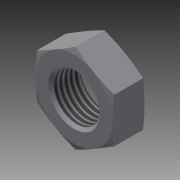
# Autodesk Inventor part: D-98
Saved by Autodesk Inventor 2014 SP2 (Build 180246200, 246)
## iProperties
Created: 2019-01-30
Part Number: D-98
Material: Generic
Catalog Web Link: www.cadenas.de
Description: Mounting Nut for Original Line Cylinders-
Vendor: BIMBA
Document SubType Name: Modeling
Designer: psadmin
Manufacturer: BIMBA
Mass: 1.65694 g
Surface Area: 11.8363 cm^2
Volume: 1.65694 cm^3
Density: 1 g/cm^3
Appearance: PSOLRGB-191-191-191
Category: PARTsolutions
Company: BIMBA
Title: D-98
Author: Cadenas PARTsolutions
PSOL_IDENT_0: {$CADENAS_DATA\23d-libs\bimba\bimba\bimba_imperial\bimba_full_line\original_line_cylinders\accessori
PSOL_IDENT_1: es\mounting_nut.prj},185 {VTYP=3D},{NB=D-98},{LINA=D-98},{NN=Mounting Nut for Original Line Cylinder
PSOL_IDENT_2: s},{DATE=27.12.2018 09:32:42},{GEOMDATE=10.11.2011 00:00:00},{VERSION=},{LINEID=60},{WBVAR=MAT},{WBN
PSOL_IDENT_3: UMERIC=}  {NB=D-98},{LINA=D-98},{KT=DUMMY},{PN=D-98},{PN1=D-98},{C=1/2-20},{TH=UNF},{MAT=},{MAT1='','
PSOL_IDENT_4: Zinc-Plated Carbon Steel', '-SS', 'Stainless Steel'},{A=0.75},{A1=0.75000000},{B=0.31},{B1=0.3100000
PSOL_IDENT_5: 0},{NDM=0.50000000},{PITCH=0.0500},{DIA=-},{DIA2=-},{DIA3=-},{DIA1=0},{DIA4=0.00000000},{DIA5=0.0000
PSOL_IDENT_6: 0000},{T=-},{T2=-},{T3=-},{T1=0},{T4=0.00000000},{T5=0.00000000},{COLOR=0.75,0.75,0.75,0.00},{TT=0.0
PSOL_IDENT_7: 5000000},{TO=0.20000000},{PRA=1}
NN: Mounting Nut for Original Line Cylinders
NB: D-98
NBSYN: $PN.
LINA: D-98
PN: D-98
C: 1/2-20
MAT: Zinc-Plated Carbon Steel
A: 0.75
B: 0.31
DIA: -
T: -
SUPPLIER: BIMBA
ARTICLENO: D-98
BOMINFO: D-98
CREATOR: CADENAS GmbH
Autodesk Inventor part; units mm, degrees
ref_plane "YZ Plane" through (0, 0, 0) normal (1, 0, 0) x (0, 1, 0)
ref_plane "XZ Plane" through (0, 0, 0) normal (0, 1, 0) x (-1, 0, 0)
ref_plane "XY Plane" through (0, 0, 0) normal (0, 0, 1) x (1, 0, 0)
sketch "Sketch_8" plane through (0, 0, 0) normal (1, 0, 0) x (0, 1, 0)
  line L0 (0, -7.874) -> (0, 0)
  line L1 (0, 0) -> (9.525, 0)
  line L2 (9.525, 0) -> (11.43, -0.5104)
  line L3 (11.43, -0.5104) -> (11.43, -7.3636)
  line L4 (11.43, -7.3636) -> (9.525, -7.874)
  line L5 (9.525, -7.874) -> (0, -7.874)
  line L6 (0, -7.874) -> (0, 0)
  constraints: 14 end point
sketch "Sketch_10" plane through (0, 0, 0) normal (0, 0, 1) x (1, 0, 0)
  line L0 (-19.05, -19.05) -> (19.05, -19.05)
  line L1 (19.05, -19.05) -> (19.05, 19.05)
  line L2 (19.05, 19.05) -> (-19.05, 19.05)
  line L3 (-19.05, 19.05) -> (-19.05, -19.05)
  line L4 (-9.525, -5.4993) -> (0, -10.9985)
  line L5 (0, -10.9985) -> (9.525, -5.4993)
  line L6 (9.525, -5.4993) -> (9.525, 5.4993)
  line L7 (9.525, 5.4993) -> (0, 10.9985)
  line L8 (0, 10.9985) -> (-9.525, 5.4993)
  line L9 (-9.525, 5.4993) -> (-9.525, -5.4993)
  constraints: 20 end point
revolve "Revolution1" add sketch "Sketch_8" angle 360 about axis through (0, 0, -7.874) along (0, 0, -1)
extrude "Extrusion1" cut sketch "Sketch_10" against normal blind 7.874
sketch "Sketch_11" plane through (0, 0, 0) normal (1, 0, 0) x (0, 1, 0)
  line L0 (0, -7.874) -> (0, 0)
  line L1 (0, 0) -> (6.35, 0)
  line L2 (6.35, 0) -> (5.6629, -0.6871)
  line L3 (5.6629, -0.6871) -> (5.6629, -7.1869)
  line L4 (5.6629, -7.1869) -> (6.35, -7.874)
  line L5 (6.35, -7.874) -> (0, -7.874)
  line L6 (0, -7.874) -> (0, 0)
  constraints: 14 end point
revolve "Revolution2" cut sketch "Sketch_11" angle 360 about axis through (0, 0, -7.874) along (0, 0, -1)
thread "Thread1" size "1/2-20 UNF" class "2B" standard "ANSI Unified Screw Threads" full length
ref_plane "NUT_XY" through (0, 0, 0) normal (0, 0, 1) x (1, 0, 0)
ref_plane "NUT_YZ" through (0, 0, 0) normal (1, 0, 0) x (0, 1, 0)
ref_plane "NUT_ZX" through (0, 0, 0) normal (0, 1, 0) x (0, 0, 1)
ref_plane "a1_XY" through (-9.525, 9.525, 0) normal (0, 0, 1) x (1, 0, 0)
ref_plane "a1_YZ" through (-9.525, 9.525, 0) normal (1, 0, 0) x (0, 1, 0)
ref_plane "a1_ZX" through (-9.525, 9.525, 0) normal (0, 1, 0) x (0, 0, 1)
ref_plane "a2_XY" through (9.525, 9.525, 0) normal (0, 0, 1) x (1, 0, 0)
ref_plane "a2_YZ" through (9.525, 9.525, 0) normal (1, 0, 0) x (0, 1, 0)
ref_plane "a2_ZX" through (9.525, 9.525, 0) normal (0, 1, 0) x (0, 0, 1)
ref_plane "b1_XY" through (0, 9.525, 0) normal (1, 0, 0) x (0, 0, -1)
ref_plane "b1_YZ" through (0, 9.525, 0) normal (0, 0, -1) x (0, 1, 0)
ref_plane "b1_ZX" through (0, 9.525, 0) normal (0, 1, 0) x (1, 0, 0)
ref_plane "b2_XY" through (0, 9.525, -7.874) normal (1, 0, 0) x (0, 0, -1)
ref_plane "b2_YZ" through (0, 9.525, -7.874) normal (0, 0, -1) x (0, 1, 0)
ref_plane "b2_ZX" through (0, 9.525, -7.874) normal (0, 1, 0) x (1, 0, 0)
ref_plane "e_XY" through (0, 0, -7.874) normal (1, 0, 0) x (0, 0, -1)
ref_plane "e_YZ" through (0, 0, -7.874) normal (0, 0, -1) x (0, 1, 0)
ref_plane "e_ZX" through (0, 0, -7.874) normal (0, 1, 0) x (1, 0, 0)
ref_plane "ol1_XY" through (0, 0, -9.525) normal (0, 1, 0) x (1, 0, 0)
ref_plane "ol1_YZ" through (0, 0, -9.525) normal (1, 0, 0) x (0, 0, -1)
ref_plane "ol1_ZX" through (0, 0, -9.525) normal (0, 0, -1) x (0, 1, 0)
ref_plane "ol2_XY" through (7.874, 0, -9.525) normal (0, 1, 0) x (1, 0, 0)
ref_plane "ol2_YZ" through (7.874, 0, -9.525) normal (1, 0, 0) x (0, 0, -1)
ref_plane "ol2_ZX" through (7.874, 0, -9.525) normal (0, 0, -1) x (0, 1, 0)
ref_plane "th1_XY" through (0, 6.35, -7.874) normal (1, 0, 0) x (0, 0, -1)
ref_plane "th1_YZ" through (0, 6.35, -7.874) normal (0, 0, -1) x (0, 1, 0)
ref_plane "th1_ZX" through (0, 6.35, -7.874) normal (0, 1, 0) x (1, 0, 0)
ref_plane "th2_XY" through (0, -6.35, -7.874) normal (1, 0, 0) x (0, 0, -1)
ref_plane "th2_YZ" through (0, -6.35, -7.874) normal (0, 0, -1) x (0, 1, 0)
ref_plane "th2_ZX" through (0, -6.35, -7.874) normal (0, 1, 0) x (1, 0, 0)
body "Solid1"
